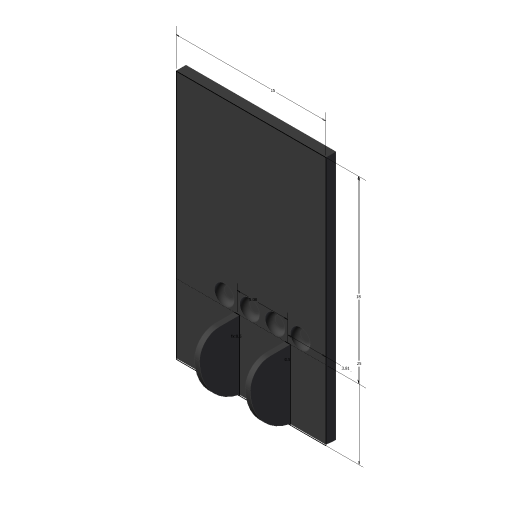
# Autodesk Inventor part: mateksys_micro_bec_support
Saved by Autodesk Inventor 2023 (Build 270158000, 158)
## iProperties
Created: 2023-02-23
Part Number: mateksys_micro_bec_support
Material: Generic
Document SubType Name: Modeling
Designer: Thomas
Density: 1 g/cm^3
Appearance: Default
Author: Thomas
Autodesk Inventor part; units mm, degrees
ref_plane "YZ Plane" through (0, 0, 0) normal (1, 0, 0) x (0, 1, 0)
ref_plane "XZ Plane" through (0, 0, 0) normal (0, 1, 0) x (-1, 0, 0)
ref_plane "XY Plane" through (0, 0, 0) normal (0, 0, 1) x (1, 0, 0)
sketch "Sketch1" plane through (0, 0, 0) normal (0, 0, 1) x (1, 0, 0)
  line L0 (0, 0) -> (15, 0)
  line L1 (15, 0) -> (15, 25)
  line L2 (15, 25) -> (0, 25)
  line L3 (0, 25) -> (0, 0)
  line L4 (0, 7) -> (15, 7) construction
  line L5 (10.94, 7) -> (11.44, 7)
  line L6 (11.44, 7) -> (11.44, 0)
  line L7 (11.44, 0) -> (10.94, 0)
  line L8 (10.94, 0) -> (10.94, 7)
  line L9 (6.36, 7) -> (5.86, 7)
  line L10 (5.86, 7) -> (5.86, 0)
  line L11 (5.86, 0) -> (6.36, 0)
  line L12 (6.36, 0) -> (6.36, 7)
  point P0 (11.19, 7)
  point P1 (6.11, 7)
  dimension "d0" = 15
  dimension "d1" = 25
  dimension "d2" = 18
  dimension "d3" = 3.81
  dimension "d4" = 0.5
  dimension "d5" = 0.5
  dimension "d6" = 5.08
  constraints: 26 end point, 6 parallel, 6 point on line, 4 horizontal, 3 perpendicular, 2 midpoint
  measures "d0" distance of L1.end L2.end
  measures "d1" distance of L0.end L1.end
  measures "d2" distance between parallel lines of L2 L4
  measures "d3" distance from line of L1 point (11.19, 7)
  measures "d4" distance between parallel lines of L6 L8
  measures "d5" distance between parallel lines of L10 L12
  measures "d6" distance of point (6.11, 7) point (11.19, 7)
extrude "Extrusion1" add sketch "Sketch1" against normal blind 1
extrude "Extrusion2" add sketch "Sketch1" along normal blind 4 contours L10 L9 L12 L0 | L8 L5 L6 L0
sketch "Sketch2" plane through (0, 0, 0) normal (0, 0, 1) x (1, 0, 0)
  line L0 (0, 7) -> (15, 7) construction
  line L1 (11.44, 7) -> (11.44, 0) projected
  line L2 (11.44, 0) -> (15, 0) projected
  line L3 (15, 0) -> (15, 25) projected
  line L4 (15, 25) -> (0, 25) projected
  line L5 (0, 25) -> (0, 0) projected
  line L6 (0, 0) -> (5.86, 0) projected
  line L7 (5.86, 0) -> (5.86, 7) projected
  line L8 (5.86, 7) -> (6.36, 7) projected
  line L9 (6.36, 7) -> (6.36, 0) projected
  line L10 (6.36, 0) -> (10.94, 0) projected
  line L11 (10.94, 0) -> (10.94, 7) projected
  line L12 (10.94, 7) -> (11.44, 7) projected
  circle A0 centre (12.46, 8) radius 1
  circle A1 centre (9.92, 8) radius 1
  circle A2 centre (7.38, 8) radius 1
  circle A3 centre (4.84, 8) radius 1
  dimension "d11" = 2
  dimension "d12" = 2.54
  dimension "d13" = 1
  dimension "d16" = 2.54
  constraints: 4 centre point, 1 horizontal, 6 other
  measures "d11" diameter of A0
  measures "d12" distance from line of A0.centre L3
  measures "d13" distance from line of A0.centre L0
  measures "d16" distance of A0.centre A1.centre
extrude "Extrusion3" cut sketch "Sketch2" against normal blind 0.5 contours A0 | A1 | A2 | A3
fillet "Fillet1" radius 0.5 4 edges at (11.46, 8, -0.5) (8.92, 8, -0.5) (6.38, 8, -0.5) (3.84, 8, -0.5)
fillet "Fillet2" radius 5 2 edges at (6.11, 0, 4) (11.19, 0, 4)
fillet "Fillet3" radius 2 2 edges at (6.11, 7, 4) (11.19, 7, 4)
equation "\"d5\" = d4"
body "Solid1"
